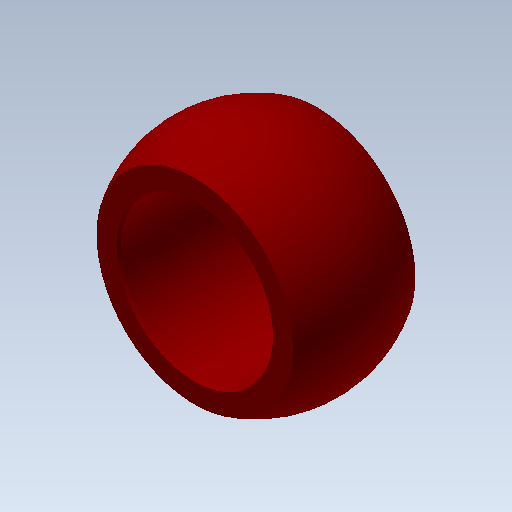
# Autodesk Inventor part: igubal Rod End Bearing Spherical Bearing
Saved by Autodesk Inventor 2020 (Build 240168000, 168)
## iProperties
Created: 2012-11-28
Document SubType Name: Modeling
Material: iglide R
Vendor: igus
Density: 1.39 g/cm^3
Description: igubal Rod End Bearing Spherical Bearing
Mass: 3.74664 g
Surface Area: 18.4052 cm^2
Volume: 2.69542 cm^3
Project: FIRST
Designer: Autodesk, Inc.
Appearance: Red - iglide R
Category: Plastic Bearings
Company: Autodesk, Inc.
Title: igubal Rod End Bearing Spherical Bearing
Author: Autodesk, Inc.
Autodesk Inventor part; units mm, degrees
ref_plane "YZ Plane" through (0, 0, 0) normal (1, 0, 0) x (0, 1, 0)
ref_plane "XZ Plane" through (0, 0, 0) normal (0, 1, 0) x (-1, 0, 0)
ref_plane "XY Plane" through (0, 0, 0) normal (0, 0, 1) x (1, 0, 0)
sketch "Sketch1" plane through (0, 0, 0) normal (0, 0, 1) x (1, 0, 0)
  arc A0 (0, -12.0015) -> (0, 12.0015) centre (0, 0) ccw
  line L0 (0, 12.0015) -> (0, -12.0015)
  line L1 (0, -16.8021) -> (0, 16.8021) projected
  dimension "d0" = 24.003
  constraints: 2 coincident, 2 end point, 2 point on circle, 1 centre point, 1 midpoint, 1 vertical
  measures "d0" diameter of A0
revolve "Revolution1" add sketch "Sketch1" angle 360 about axis through (0, -10, 0) along (0, 1, 0)
sketch "Sketch4" plane through (0, 0, 0) normal (1, 0, 0) x (0, 1, 0)
  circle A0 centre (0, 0) radius 12.0015 projected
  line L0 (-10.184, 6.35) -> (10.184, 6.35)
  line L1 (0, 6.35) -> (0, 0)
  line L2 (0, 0) -> (0, -6.35)
  line L3 (-10.184, -6.35) -> (10.184, -6.35)
  dimension "d8" = 12.7
  constraints: 8 end point, 4 point on circle, 2 collinear, 2 midpoint, 2 perpendicular, 1 horizontal
  measures "d8" distance between parallel lines of L3 L0
extrude "Extrusion3" cut sketch "Sketch4" along normal through all both and the other way through all contours A0 L3 L2 L1 L0 | L0 L1 L2 L3 A0 keep common part
hole "Hole1" at (0, 0, 6.35) direction (0, 0, -1) diameter 15.875 end through all
chamfer "Chamfer1" distance 0.3048 angle 30 1 edges at (0, 7.9375, 6.35) measured on face at (0, 7.9375, 5.85)
body "Solid1"
